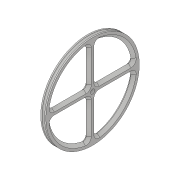
# Autodesk Inventor part: Wheel
Saved by Autodesk Inventor 2017 (Build 210142000, 142)
## iProperties
Created: 2019-06-10
Part Number: Wheel
Material: Generic
Document SubType Name: Modeling
Designer: markg
Density: 1 g/cm^3
Appearance: Default
Author: markg
Autodesk Inventor part; units mm, degrees
ref_plane "YZ Plane" through (0, 0, 0) normal (1, 0, 0) x (0, 1, 0)
ref_plane "XZ Plane" through (0, 0, 0) normal (0, 1, 0) x (-1, 0, 0)
ref_plane "XY Plane" through (0, 0, 0) normal (0, 0, 1) x (1, 0, 0)
sketch "Sketch1" plane through (0, 0, 0) normal (0, 1, 0) x (-1, 0, 0)
  line L0 (0, 0) -> (-6.35, 0)
  line L1 (-6.35, 0) -> (-6.35, -57.15)
  line L2 (0, -57.15) -> (0, 0)
  arc A0 (-1.5875, -57.15) -> (-4.7625, -57.15) centre (-3.175, -57.15) ccw
  line L3 (-6.35, -57.15) -> (-4.7625, -57.15)
  line L4 (-1.5875, -57.15) -> (0, -57.15)
  dimension "d0" = 6.35
  dimension "d1" = 57.15
  dimension "d2" = 3.175
  constraints: 10 end point, 3 parallel, 2 point on circle, 1 centre point, 1 horizontal, 1 perpendicular
  measures "d0" distance of L2.start L1.end
  measures "d1" distance of L1.end L0.end
  measures "d2" diameter of A0
revolve "Revolution1" add sketch "Sketch1" angle 360 about axis through (0, 0, 0) along (1, 0, 0)
sketch "Sketch2" plane through (6.35, 0, 0) normal (1, 0, 0) x (0, 0, -1)
  line L0 (-4.7625, 50.5763) -> (-4.7625, 4.7625)
  line L1 (-4.7625, -4.7625) -> (-4.7625, -50.5763)
  line L2 (4.7625, 50.5763) -> (4.7625, 4.7625)
  line L3 (4.7625, -4.7625) -> (4.7625, -50.5763)
  arc A0 (50.5763, 4.7625) -> (4.7625, 50.5763) centre (0, 0) ccw
  arc A1 (-4.7625, 50.5763) -> (-50.5763, 4.7625) centre (0, 0) ccw
  line L4 (-50.5763, 4.7625) -> (-4.7625, 4.7625)
  line L5 (4.7625, 4.7625) -> (50.5763, 4.7625)
  line L6 (-50.5763, -4.7625) -> (-4.7625, -4.7625)
  line L7 (4.7625, -4.7625) -> (50.5763, -4.7625)
  arc A2 (-50.5763, -4.7625) -> (-4.7625, -50.5763) centre (0, 0) ccw
  arc A3 (4.7625, -50.5763) -> (50.5763, -4.7625) centre (0, 0) ccw
  constraints: 16 end point, 8 parallel, 8 point on circle, 4 centre point, 2 horizontal, 2 vertical, 1 coincident
extrude "Extrusion1" cut sketch "Sketch2" against normal blind 25.4
fillet "Fillet1" radius 3.175 12 edges at (3.175, 4.7625, 4.7625) (3.175, 4.7625, -4.7625) (3.175, -4.7625, -4.7625) (3.175, -4.7625, 4.7625) (3.175, -4.7625, -50.5763) (3.175, -50.5763, -4.7625) (3.175, -50.5763, 4.7625) (3.175, -4.7625, 50.5763) (3.175, 4.7625, 50.5763) (3.175, 50.5763, 4.7625) (3.175, 50.5763, -4.7625) (3.175, 4.7625, -50.5763)
sketch "Sketch3" plane through (6.35, 0, 0) normal (1, 0, 0) x (0, 0, -1)
  circle A0 centre (0, 0) radius 2.54
  dimension "d12" = 5.08
  constraints: 1 centre point, 1 coincident
  measures "d12" diameter of A0
extrude "Extrusion2" cut sketch "Sketch3" against normal blind 25.4
chamfer "Chamfer1" distance 3.175 angle 45 48 edges at (6.35, -27.4482, -4.7625) (6.35, -5.6924, -5.6924) (6.35, -4.7625, -27.4482) (6.35, -5.888, -49.3838) (6.35, -35.921, -35.921) (6.35, -49.3838, -5.888) (6.35, -27.4482, 4.7625) (6.35, -49.3838, 5.888) (6.35, -35.921, 35.921) (6.35, -5.888, 49.3838) (6.35, -4.7625, 27.4482) (6.35, -5.6924, 5.6924) (6.35, 5.6924, 5.6924) (6.35, 27.4482, 4.7625) (6.35, 49.3838, 5.888) (6.35, 35.921, 35.921) (6.35, 5.888, 49.3838) (6.35, 4.7625, 27.4482) (6.35, 5.6924, -5.6924) (6.35, 4.7625, -27.4482) (6.35, 5.888, -49.3838) (6.35, 35.921, -35.921) (6.35, 49.3838, -5.888) (6.35, 27.4482, -4.7625) (0, 5.6924, 5.6924) (0, 4.7625, 27.4482) (0, 5.888, 49.3838) (0, 35.921, 35.921) (0, 49.3838, 5.888) (0, 27.4482, 4.7625) (0, -5.6924, 5.6924) (0, -27.4482, 4.7625) (0, -49.3838, 5.888) (0, -35.921, 35.921) (0, -5.888, 49.3838) (0, -4.7625, 27.4482) (0, -5.6924, -5.6924) (0, -4.7625, -27.4482) (0, -5.888, -49.3838) (0, -35.921, -35.921) (0, -49.3838, -5.888) (0, -27.4482, -4.7625) (0, 5.6924, -5.6924) (0, 27.4482, -4.7625) (0, 49.3838, -5.888) (0, 35.921, -35.921) (0, 5.888, -49.3838) (0, 4.7625, -27.4482)
body "Solid1"
